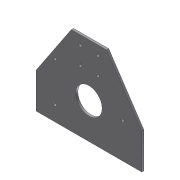
# Autodesk Inventor part: Plate_PictureMountPlate
Saved by Autodesk Inventor 2012 (Build 160160000, 160)
## iProperties
Created: 2012-01-19
Part Number: Plate_PictureMountPlate
Material: Default
Document SubType Name: Modeling
Designer: JesseK
Density: 1 g/cm^3
Mass: 45.1455 g
Surface Area: 306.999 cm^2
Volume: 45.1455 cm^3
Author: JesseK
Autodesk Inventor part; units mm, degrees
ref_plane "YZ Plane" through (0, 0, 0) normal (1, 0, 0) x (0, 1, 0)
ref_plane "XZ Plane" through (0, 0, 0) normal (0, 1, 0) x (-1, 0, 0)
ref_plane "XY Plane" through (0, 0, 0) normal (0, 0, 1) x (1, 0, 0)
sketch "Sketch1" plane through (0, 0, 0) normal (0, 0, 1) x (1, 0, 0)
  line L0 (0, 50.8) -> (-50.8, 50.8)
  line L1 (-101.6, -76.2) -> (50.8, -76.2)
  line L2 (0, 0) -> (0, 50.8) construction
  line L3 (-101.6, -76.2) -> (-101.6, -25.4)
  line L4 (-101.6, -25.4) -> (-50.8, 50.8)
  line L5 (0, 50.8) -> (50.8, -25.4)
  line L6 (50.8, -25.4) -> (50.8, -76.2)
  dimension "d0" = 50.8
  dimension "d3" = 50.8
  dimension "d17" = 127
  dimension "d18" = 50.8
  dimension "d26" = 152.4
  constraints: 14 end point, 3 vertical, 2 equal length, 1 horizontal, 1 parallel
  measures "d0" distance of L0.start L0.end
  measures "d3" distance of L2.start L0.start
  measures "d17" distance between parallel lines of L0 L1
  measures "d18" distance of L1.start L3.end
  measures "d26" distance of L1.start L1.end
extrude "Extrusion1" add sketch "Sketch1" along normal blind 3.175
sketch "Sketch2" plane through (0, 0, 3.175) normal (0, 0, 1) x (1, 0, 0)
  line L0 (-50.8, 50.8) -> (0, 50.8) projected
  line L1 (-50.8, -76.2) -> (-50.8, 50.8) projected
  circle A0 centre (-38.1, 38.1) radius 2.3813
  circle A1 centre (-12.7, 38.1) radius 2.3813
  circle A2 centre (-38.1, 12.7) radius 2.3813
  circle A3 centre (-12.7, 12.7) radius 2.3813
  line L2 (-38.1, 38.1) -> (-12.7, 38.1) construction
  line L3 (-12.7, 38.1) -> (-12.7, 12.7) construction
  line L4 (-12.7, 12.7) -> (-38.1, 12.7) construction
  line L5 (-38.1, 12.7) -> (-38.1, 38.1) construction
  point P0 (-101.6, -76.2)
  point P1 (0, 0)
  dimension "d6" = 4.7625
  dimension "d7" = 12.7
  dimension "d8" = 25.4
  dimension "d9" = 12.7
  dimension "d10" = 25.4
  constraints: 8 end point, 4 centre point, 3 equal radius, 2 coincident, 2 parallel, 1 horizontal, 1 perpendicular, 1 other
  measures "d6" diameter of A2
  measures "d8" distance of L2.start L2.end
  measures "d9" distance between parallel lines of L0 L2
  measures "d10" distance of L4.end L2.start
extrude "Extrusion2" cut sketch "Sketch2" against normal up to next
sketch "Sketch3" plane through (0, 0, 3.175) normal (0, 0, 1) x (1, 0, 0)
  circle A0 centre (-25.4, -25.4) radius 19.05
  point P0 (0, 0)
  dimension "d13" = 25.4
  dimension "d14" = 38.1
  constraints: 1 centre point
  measures "d13" horizontal distance of point (0, 0) A0.centre
  measures "d14" diameter of A0
extrude "Extrusion3" cut sketch "Sketch3" against normal up to next
sketch "Sketch4" plane through (0, 0, 3.175) normal (0, 0, 1) x (1, 0, 0)
  circle A0 centre (-74.4647, 2.9021) radius 2.3813
  circle A1 centre (-74.4647, -54.2479) radius 2.3813
  circle A2 centre (22.9075, -25.1429) radius 2.3813
  line L0 (-74.4647, 2.9021) -> (-74.4647, -54.2479)
  point P0 (0, 0)
  dimension "d20" = 4.7625
  dimension "d23" = 57.15
  constraints: 3 centre point, 2 end point, 2 equal radius, 1 vertical
  measures "d20" diameter of A0
  measures "d23" distance of L0.start L0.end
extrude "Extrusion4" cut sketch "Sketch4" against normal up to next
body "Solid1"
